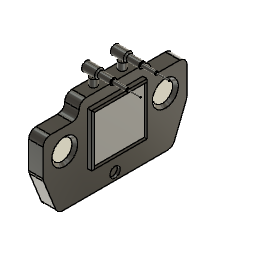
Radio Controller (Autodesk Fusion 360 design; units mm, degrees)
Autodesk Fusion 360 part; units mm, degrees
note: some values were not read from the file. Chosen so that the rebuilt part matches the saved one: where a step ends. Set by a fixed rule: which sketch regions a step uses.
sketch "Sketch1" plane through (0, 0, 0) normal (1, 0, 0) x (0, 1, 0)
  line L0 (0, 0) -> (0, 50)
  line L1 (0, 50) -> (25, 50)
  line L2 (25, 50) -> (25, 60)
  line L3 (25, 60) -> (75, 60)
  line L4 (75, 60) -> (75, 50)
  line L5 (100, 50) -> (100, 0)
  line L6 (100, 0) -> (0, 0)
  line L7 (75, 50) -> (100, 50)
  line L8 (0, 25) -> (100, 25)
  dimension "d2" = 50
  dimension "d3" = 25
  dimension "d4" = 75
  dimension "d5" = 100
  dimension "d6" = 10
  dimension "d7" = 60
  constraint coincident L0.start L6.end
  constraint vertical L0
  constraint perpendicular L0 L1
  constraint perpendicular L1 L2
  constraint perpendicular L2 L3
  constraint perpendicular L1 L4
  constraint perpendicular L1 L5
  constraint perpendicular L0 L6
  constraint perpendicular L5 L7
  constraint midpoint L0 L8.start
  constraint midpoint L5 L8.end
  measures "d2" distance of L5.start L5.end
  measures "d3" horizontal distance of L0.start L2.end
  measures "d4" horizontal distance of L0.start L3.end
  measures "d5" horizontal distance of L0.start L5.start
  measures "d6" distance of L1.end L2.end
  measures "d7" distance of L3 L6
extrude "Extrude1" add sketch "Sketch1" along normal blind 10 contours L0 L1 L2 L3 L4 L5 L7 L8 makes body 1
extrude "Extrude2" add sketch "Sketch1" along normal blind 10 contours L0 L5 L6 L8 bodies 1
fillet "Fillet1" radius 5 4 edges at (5, 0, 50) (5, 25, 60) (5, 75, 60) (5, 100, 50) on bodies 1
fillet "Fillet2" radius 5 2 edges at (5, 25, 50) (5, 75, 50) on bodies 1
sketch "Sketch2" plane through (0, 100, 0) normal (0, 1, 0) x (-1, 0, 0)
  line L0 (0, 45) -> (-10, 45)
  line L1 (-10, 45) -> (-10, 0)
  line L2 (-10, 0) -> (0, 0)
  line L3 (0, 0) -> (0, 45)
  line L4 (0, 25) -> (-10, 25)
  constraint coincident L3 L4.start
  constraint coincident L1 L4.end
  constraint perpendicular L1 L4
sketch "Sketch3" plane through (10, 0, 0) normal (1, 0, 0) x (0, 1, 0)
  arc A0 (100, 45) -> (95, 50) centre (95, 45) ccw
  line L0 (95, 50) -> (80, 50)
  arc A1 (75, 55) -> (80, 50) centre (80, 55) ccw
  arc A2 (75, 55) -> (70, 60) centre (70, 55) ccw
  line L1 (70, 60) -> (30, 60)
  arc A3 (30, 60) -> (25, 55) centre (30, 55) ccw
  arc A4 (20, 50) -> (25, 55) centre (20, 55) ccw
  line L2 (20, 50) -> (5, 50)
  arc A5 (5, 50) -> (0, 45) centre (5, 45) ccw
  line L3 (0, 45) -> (0, 0)
  line L4 (0, 0) -> (100, 0)
  line L5 (100, 0) -> (100, 45)
  line L6 (100, 25) -> (0, 25)
  constraint coincident L5 L6.start
  constraint coincident L3 L6.end
  constraint perpendicular L3 L6
sketch "Sketch4" plane through (0, 100, 0) normal (0, 1, 0) x (-1, 0, 0)
  line L0 (0, 25) -> (-10, 25)
  constraint horizontal L0
sketch "Sketch5" plane through (0, 100, 0) normal (0, 1, 0) x (-1, 0, 0)
  line L0 (0, 25) -> (-10, 25)
  constraint horizontal L0
sketch "Sketch6" plane through (0, 0, 0) normal (0, 1, 0) x (1, 0, 0)
  line L0 (0, -25) -> (10, -25)
  constraint horizontal L0
chamfer "Chamfer1" distance 10 distance2 25 1 edges at (5, 100, 0) measured on face at (3.3333, 66.6667, 0) on bodies 1
chamfer "Chamfer2" distance 25 distance2 10 1 edges at (5, 0, 0) measured on face at (3.3333, 0, 15) on bodies 1
fillet "Fillet3" radius 5 1 edges at (5, 10, 0) on bodies 1
fillet "Fillet4" radius 5 1 edges at (5, 90, 0) on bodies 1
fillet "Fillet5" radius 5 2 edges at (5, 100, 25) (5, 0, 25) on bodies 1
sketch "Sketch7" plane through (10, 0, 0) normal (1, 0, 0) x (0, 1, 0)
  circle A0 centre (15, 35) radius 7
  circle A1 centre (85, 35) radius 7
  line L0 (30.703, 53.1563) -> (69.297, 53.1563)
  line L1 (69.297, 53.1563) -> (69.297, 16.8437)
  line L2 (69.297, 16.8437) -> (30.703, 16.8437)
  line L3 (30.703, 16.8437) -> (30.703, 53.1563)
  line L4 (30.703, 53.1563) -> (69.297, 16.8437) construction
  line L5 (69.297, 53.1563) -> (30.703, 16.8437) construction
  dimension "d26" = 14
  dimension "d27" = 14
  constraint horizontal L0
  constraint perpendicular L0 L1
  constraint parallel L0 L2
  constraint parallel L1 L3
  measures "d26" diameter of A0
  measures "d27" diameter of A1
extrude "Extrude3" cut sketch "Sketch7" against normal blind 2 contours A0 bodies 1
extrude "Extrude4" cut sketch "Sketch7" against normal blind 2 contours A1 bodies 1
chamfer "Chamfer3" distance 2 distance2 2 2 edges at (10, 78.4737, 37.5313) (10, 8.4737, 37.5313) measured on face at (10, 59.7388, 10.3523) measured on face at (10, 59.7388, 10.3523) on bodies 1
extrude "Extrude5" cut sketch "Sketch7" against normal blind 1 contours L0 L1 L2 L3 bodies 1
sketch "Sketch8" plane through (10, 0, 0) normal (1, 0, 0) x (0, 1, 0)
  circle A0 centre (50, 5) radius 3.57
  dimension "d36" = 7.1401
  measures "d36" diameter of A0
extrude "Extrude6" cut sketch "Sketch8" against normal blind 2 bodies 1
sketch "Sketch9" plane through (0, 0, 60) normal (0, 0, 1) x (-1, 0, 0)
  line L0 (-10, -70) -> (0, -70)
  line L1 (0, -70) -> (0, -30)
  line L2 (0, -30) -> (-10, -30)
  line L3 (-10, -30) -> (-10, -70)
  line L4 (-5, -70) -> (-5, -30)
  circle A0 centre (-5, -60) radius 2.5
  circle A1 centre (-5, -40) radius 2.5
  dimension "d39" = 5
  dimension "d40" = 5
  constraint midpoint L0 L4.start
  constraint perpendicular L0 L4
  constraint coincident L4 A0.centre
  constraint coincident L4 A1.centre
  measures "d39" diameter of A0
  measures "d40" diameter of A1
sketch "Sketch10" plane through (0, 0, 60) normal (0, 0, 1) x (-1, 0, 0)
extrude "Extrude7" add sketch "Sketch9" along normal blind 5 contours L4 A0 | L4 A0 | L4 A1 | L4 A1 bodies 1
ref_plane "WorkPlane1" through (5, 50, 30) normal (1, 0, 0) x (0, 0, -1)
sketch "Sketch11" plane through (0, 0, 0) normal (1, 0, 0) x (0, 1, 0)
  circle A0 centre (40, 69) radius 3.25
  circle A1 centre (60, 69) radius 3.25
  circle A2 centre (40, 69) radius 2.25
  circle A3 centre (60, 69) radius 2.25
  circle A4 centre (40, 69) radius 1.25
  circle A5 centre (60, 69) radius 1.25
  circle A6 centre (40, 69) radius 0.5
  circle A7 centre (60, 69) radius 0.5
  line L0 (39.0883, 65.8805) -> (39.0883, 65)
  line L1 (40.9117, 65.8805) -> (40.9117, 65)
  line L2 (59.0883, 65.8805) -> (59.0883, 65)
  line L3 (60.9117, 65.8805) -> (60.9117, 65)
  dimension "d44" = 6.5
  dimension "d45" = 6.5
  dimension "d46" = 4.5
  dimension "d47" = 4.5
  dimension "d48" = 2.5
  dimension "d49" = 2.5
  dimension "d50" = 1
  dimension "d51" = 1
  constraint concentric A0 A2
  constraint concentric A1 A3
  constraint concentric A2 A4
  constraint concentric A3 A5
  constraint concentric A2 A6
  constraint concentric A5 A7
  constraint coincident A0 L0.start
  constraint vertical L0
  constraint coincident A0 L1.start
  constraint parallel L0 L1
  constraint coincident A1 L2.start
  constraint parallel L1 L2
  constraint coincident A1 L3.start
  constraint parallel L2 L3
  measures "d44" diameter of A0
  measures "d45" diameter of A1
  measures "d46" diameter of A2
  measures "d47" diameter of A3
  measures "d48" diameter of A4
  measures "d49" diameter of A5
  measures "d50" diameter of A6
  measures "d51" diameter of A7
extrude "Extrude8" add sketch "Sketch11" along normal blind 10 separate body contours A0 | A1 makes body 2 at (6.6667, 43.2339, 69.3236) makes body 3 at (6.6667, 57.5104, 71.0891)
extrude "Extrude9" add sketch "Sketch11" along normal blind 19 contours A2 | A3 bodies 2 3
extrude "Extrude10" add sketch "Sketch11" along normal blind 29 contours A4 | A5 bodies 2 3
extrude "Extrude11" add sketch "Sketch11" along normal blind 38 contours A6 | A7 bodies 2 3
sketch "Sketch12" plane through (0, 0, 0) normal (1, 0, 0) x (0, 1, 0)
  line L0 (39, 65) -> (41, 65)
  line L1 (59, 65) -> (61, 65)
  constraint horizontal L0
  constraint horizontal L1
sketch "Sketch13" plane through (0, 0, 0) normal (1, 0, 0) x (0, 1, 0)
sketch "Sketch14" plane through (0, 0, 65) normal (0, 0, 1) x (-1, 0, 0)
  circle A0 centre (-5, -40) radius 2.5
  circle A1 centre (-5, -40) radius 0.6252
  circle A2 centre (-5, -60) radius 0.625
  dimension "d60" = 1.2504
  dimension "d61" = 1.25
  constraint concentric A0 A1
  measures "d60" diameter of A1
  measures "d61" diameter of A2
extrude "Extrude12" add sketch "Sketch14" along normal up to far side of body 3 contours A2 bodies 3 1
sketch "Sketch15" plane through (0, 0, 65) normal (0, 0, 1) x (-1, 0, 0)
  circle A0 centre (-5, -40) radius 2.5
  circle A1 centre (-5, -40) radius 0.625
  dimension "d63" = 1.25
  constraint concentric A0 A1
  measures "d63" diameter of A1
extrude "Extrude13" add sketch "Sketch15" along normal up to far side of body 2 contours A1 bodies 2 3
chamfer "Chamfer4" distance 1 angle 45 2 edges at (10, 36.9699, 67.8248) (10, 56.9699, 67.8248) on bodies 2
chamfer "Chamfer5" distance 0.3 angle 45 6 edges at (19, 37.9023, 68.1864) (19, 57.9023, 68.1864) (29, 58.8346, 68.548) (29, 38.8346, 68.548) (38, 39.5338, 68.8192) (38, 59.5338, 68.8192) on bodies 2
sketch "Sketch16" plane through (9, 0, 0) normal (1, 0, 0) x (0, 1, 0)
  line L0 (30.703, 16.8437) -> (69.297, 16.8437)
  line L1 (69.297, 16.8437) -> (69.297, 53.1563)
  line L2 (69.297, 53.1563) -> (30.703, 53.1563)
  line L3 (30.703, 53.1563) -> (30.703, 16.8437)
extrude "Extrude14" add sketch "Sketch16" along normal blind 5 bodies 2
chamfer "Chamfer6" distance 1 angle 45 4 edges at (14, 30.703, 35) (14, 50, 53.1563) (14, 69.297, 35) (14, 50, 16.8437) on bodies 2
extrude "Extrude15" cut 1 faces at (14, 43.901, 29.2812) along direction (-1, 0, 0) blind 2 on bodies 2 bodies 2
